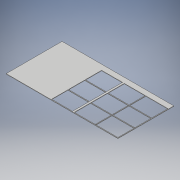
# Autodesk Inventor part: Test_Panel
Saved by Autodesk Inventor 2019.4 (Build 234330000, 330)
## iProperties
Created: 2020-02-07
Part Number: Test_Panel
Material: Generic
Document SubType Name: Modeling
Designer: Jorian Bruslind
Density: 1 g/cm^3
Appearance: Default
Author: Jorian Bruslind
Autodesk Inventor part; units mm, degrees
ref_plane "YZ Plane" through (0, 0, 0) normal (1, 0, 0) x (0, 1, 0)
ref_plane "XZ Plane" through (0, 0, 0) normal (0, 1, 0) x (-1, 0, 0)
ref_plane "XY Plane" through (0, 0, 0) normal (0, 0, 1) x (1, 0, 0)
sketch "Sketch1" plane through (0, 0, 0) normal (0, 1, 0) x (-1, 0, 0)
  line L0 (0, 0) -> (-2438.4, 0)
  line L1 (-2438.4, 0) -> (-2438.4, -1219.2)
  line L2 (-2438.4, -1219.2) -> (0, -1219.2)
  line L3 (0, -1219.2) -> (0, 0)
  line L4 (-2438.4, 0) -> (-2438.4, -12.7)
  line L5 (-2438.4, -12.7) -> (-2425.7, -12.7)
  line L6 (-2425.7, -12.7) -> (-1943.1, -12.7)
  line L7 (-1943.1, -12.7) -> (-1943.1, -368.3)
  line L8 (-1943.1, -368.3) -> (-2425.7, -368.3)
  line L9 (-2425.7, -368.3) -> (-2425.7, -12.7)
  line L10 (-1943.1, -381) -> (-1943.1, -736.6)
  line L11 (-1943.1, -736.6) -> (-2425.7, -736.6)
  line L12 (-2425.7, -736.6) -> (-2425.7, -381)
  line L13 (-2425.7, -381) -> (-1943.1, -381)
  line L14 (-1943.1, -749.3) -> (-1943.1, -1104.9)
  line L15 (-1943.1, -1104.9) -> (-2425.7, -1104.9)
  line L16 (-2425.7, -1104.9) -> (-2425.7, -749.3)
  line L17 (-2425.7, -749.3) -> (-1943.1, -749.3)
  line L18 (-1943.1, -12.7) -> (-1930.4, -12.7)
  line L19 (-1930.4, -12.7) -> (-1473.2, -12.7)
  line L20 (-1473.2, -12.7) -> (-1473.2, -368.3)
  line L21 (-1473.2, -368.3) -> (-1930.4, -368.3)
  line L22 (-1930.4, -368.3) -> (-1930.4, -12.7)
  line L23 (-1473.2, -736.6) -> (-1930.4, -736.6)
  line L24 (-1930.4, -736.6) -> (-1930.4, -381)
  line L25 (-1930.4, -381) -> (-1473.2, -381)
  line L26 (-1473.2, -381) -> (-1473.2, -736.6)
  line L27 (-1473.2, -1104.9) -> (-1930.4, -1104.9)
  line L28 (-1930.4, -1104.9) -> (-1930.4, -749.3)
  line L29 (-1930.4, -749.3) -> (-1473.2, -749.3)
  line L30 (-1473.2, -749.3) -> (-1473.2, -1104.9)
  line L31 (-977.9, -368.3) -> (-1435.1, -368.3)
  line L32 (-1435.1, -368.3) -> (-1435.1, -12.7)
  line L33 (-1435.1, -12.7) -> (-977.9, -12.7)
  line L34 (-977.9, -12.7) -> (-977.9, -368.3)
  line L35 (-977.9, -736.6) -> (-1435.1, -736.6)
  line L36 (-1435.1, -736.6) -> (-1435.1, -381)
  line L37 (-1435.1, -381) -> (-977.9, -381)
  line L38 (-977.9, -381) -> (-977.9, -736.6)
  line L39 (-977.9, -1104.9) -> (-1435.1, -1104.9)
  line L40 (-1435.1, -1104.9) -> (-1435.1, -749.3)
  line L41 (-1435.1, -749.3) -> (-977.9, -749.3)
  line L42 (-977.9, -749.3) -> (-977.9, -1104.9)
  dimension "d0" = 2438.4
  dimension "d1" = 1219.2
  dimension "d2" = 12.7
  dimension "d3" = 12.7
  dimension "d4" = 482.6
  dimension "d5" = 355.6
  dimension "d8" = 368.3
  dimension "d13" = 12.7
  dimension "d14" = 457.2
  dimension "d15" = 355.6
  dimension "d18" = 368.3
  dimension "d21" = 495.3
  constraints: 86 end point, 6 horizontal, 6 parallel, 3 perpendicular, 2 vertical, 1 point on line, 56 other
  measures "d0" distance of L2.end L1.end
  measures "d1" distance of L1.end L0.end
  measures "d2" distance of L0.end L4.end
  measures "d3" distance of L4.end L5.end
  measures "d4" distance of L7.end L8.end
  measures "d5" distance of L6.end L7.end
  measures "d8" distance of L6.end L10.start
  measures "d13" distance of L6.end L18.end
  measures "d14" distance of L20.end L21.end
  measures "d15" distance of L19.end L20.end
  measures "d18" distance of L20.end L23.start
  measures "d21" distance of L20.end L31.start
extrude "Extrusion1" add sketch "Sketch1" along normal blind 10
body "Solid1"
